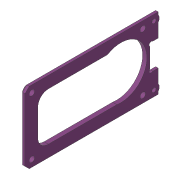
# Autodesk Inventor part: SERVO_BOTTOM_SPACER
Saved by Autodesk Inventor 2019.4 (Build 234330000, 330)
## iProperties
Created: 2019-11-13
Part Number: SERVO_BOTTOM_SPACER
Material: 一般
Document SubType Name: Modeling
Designer: y6tada
Density: 1 g/cm^3
Appearance: 滑らか - 紫
Author: y6tada
Autodesk Inventor part; units mm, degrees
ref_plane "YZ Plane" through (0, 0, 0) normal (1, 0, 0) x (0, 1, 0)
ref_plane "XZ Plane" through (0, 0, 0) normal (0, 1, 0) x (-1, 0, 0)
ref_plane "XY Plane" through (0, 0, 0) normal (0, 0, 1) x (1, 0, 0)
sketch "スケッチ1" plane through (0, 0, 0) normal (1, 0, 0) x (0, 1, 0)
  line L0 (0, 0) -> (0, 58.5) construction
  line L1 (16.75, 56.5) -> (16.75, -4)
  line L2 (16.75, -4) -> (15.5, -4)
  line L3 (6.1, -4) -> (6.1, -1.4142)
  line L4 (5.714, 0) -> (4.6858, 0) construction
  line L5 (4.6858, 0) -> (-4.6858, 0)
  line L6 (-6.1, 0) -> (-6.1, -1.4142) construction
  line L7 (-6.1, -4) -> (-12.5, -4)
  line L8 (-16.75, -4) -> (-16.75, 56.5)
  arc A0 (-4.6858, 0) -> (-6.1, -1.4142) centre (-5.3929, -0.7071) ccw
  line L9 (14.75, 58.5) -> (-14.75, 58.5)
  line L10 (16.75, 56.5) -> (14.75, 58.5)
  line L11 (-16.75, 56.5) -> (-14.75, 58.5)
  line L12 (13.5, 55.25) -> (-13.5, 55.25) construction
  line L13 (-13.5, 55.25) -> (-13.5, 3.25) construction
  line L14 (-13.5, 3.25) -> (13.5, 3.25) construction
  line L15 (13.5, 3.25) -> (13.5, 55.25) construction
  line L16 (0, 29.25) -> (21.0927, 29.25) construction
  line L17 (14, -2) -> (-14, -2) construction
  arc A1 (12.5, -4) -> (15.5, -4) centre (14, -2) ccw
  line L18 (15.5, -4) -> (12.5, -4) construction
  line L19 (12.5, -4) -> (6.1, -4)
  arc A2 (-15.5, -4) -> (-12.5, -4) centre (-14, -2) ccw
  line L20 (-12.5, -4) -> (-15.5, -4) construction
  line L21 (-15.5, -4) -> (-16.75, -4)
  line L22 (6.25, 52.5) -> (-6.25, 52.5)
  line L23 (-11.25, 47.5) -> (-11.25, 12)
  line L24 (-11.25, 12) -> (11.25, 12)
  line L25 (11.25, 12) -> (11.25, 47.5)
  arc A3 (11.25, 47.5) -> (6.25, 52.5) centre (6.25, 47.5) ccw
  arc A4 (-6.25, 52.5) -> (-11.25, 47.5) centre (-6.25, 47.5) ccw
  line L26 (6.1, -1.4142) -> (6.1, -0.7071) construction
  line L27 (-4.6858, 0) -> (-6.1, 0) construction
  line L28 (-6.1, -1.4142) -> (-6.1, -4)
  line L29 (6.1, -1.4142) -> (6.1, 0) construction
  line L30 (6.1, 0) -> (4.6858, 0) construction
  arc A5 (6.1, -1.4142) -> (4.6858, 0) centre (5.3929, -0.7071) ccw
  point P0 (16.75, 58.5)
  point P1 (-6.0944, 0.0056)
  point P2 (-16.75, 58.5)
  dimension "d3" = 12.2
  dimension "d5" = 33.5
  dimension "d6" = 4
  dimension "d7" = 58.5
  dimension "d8" = 2
  dimension "d9" = 2
  dimension "d10" = 2
  dimension "d11" = 2
  dimension "d12" = 27
  dimension "d13" = 52
  dimension "d14" = 2
  dimension "d15" = 28
  dimension "d16" = 2.5
  dimension "d33" = 5
  dimension "d34" = 5.5
  dimension "d35" = 6
  dimension "d36" = 12
  dimension "d37" = 1
  constraints: 62 end point, 16 perpendicular, 15 point on circle, 8 point on line, 7 coincident, 6 centre point, 6 horizontal, 4 parallel, 4 symmetric about line, 4 tangent, 4 vertical, 3 midpoint, 2 equal radius, 1 collinear, 6 other
  measures "d3" distance between parallel lines of L6 L3
  measures "d5" distance between parallel lines of L8 L1
  measures "d6" distance between parallel lines of L2 L5
  measures "d7" distance from line of L9 L0.start
  measures "d8" distance of L1.start point (16.75, 58.5)
  measures "d9" distance of L9.start point (16.75, 58.5)
  measures "d10" distance of L8.end point (-16.75, 58.5)
  measures "d11" distance of L9.end point (-16.75, 58.5)
  measures "d12" distance of L12.start L12.end
  measures "d13" distance of L14.end L12.start
  measures "d14" distance between parallel lines of L5 L17
  measures "d15" distance of L17.start L17.end
  measures "d16" radius of A1
  measures "d33" radius of A3
  measures "d34" distance between parallel lines of L1 L25
  measures "d35" distance between parallel lines of L9 L22
  measures "d36" distance between parallel lines of L5 L24
  measures "d37" radius of A5
extrude "押し出し1" add sketch "スケッチ1" against normal blind 1.2
sketch "スケッチ2" plane through (-1.2, 0, 0) normal (1, 0, 0) x (0, 0, -1)
  line L0 (-58.5, 14.75) -> (-58.5, -14.75) construction
  line L1 (-56.5, -16.75) -> (4, -16.75) construction
  line L2 (4, 16.75) -> (-56.5, 16.75) construction
  line L3 (0, -4.6858) -> (0, 4.6858) construction
  line L4 (-0.8, 13.9287) -> (-0.8, -13.9287)
  line L5 (-2.8213, -15.95) -> (-55.6787, -15.95)
  line L6 (-57.7, -13.9287) -> (-57.7, 13.9287)
  line L7 (-55.6787, 15.95) -> (-2.8213, 15.95)
  line L8 (-1.2393, -14.9893) -> (-1.7607, -15.5107)
  line L9 (-1.2393, 14.9893) -> (-1.7607, 15.5107)
  line L10 (-56.7393, 15.5107) -> (-57.2607, 14.9893)
  line L11 (-57.2607, -14.9893) -> (-56.7393, -15.5107)
  arc A0 (-1.2393, -14.9893) -> (-0.8, -13.9287) centre (-2.3, -13.9287) ccw
  arc A1 (-2.8213, -15.95) -> (-1.7607, -15.5107) centre (-2.8213, -14.45) ccw
  arc A2 (-56.7393, -15.5107) -> (-55.6787, -15.95) centre (-55.6787, -14.45) ccw
  arc A3 (-57.7, -13.9287) -> (-57.2607, -14.9893) centre (-56.2, -13.9287) ccw
  arc A4 (-55.6787, 15.95) -> (-56.7393, 15.5107) centre (-55.6787, 14.45) ccw
  arc A5 (-57.2607, 14.9893) -> (-57.7, 13.9287) centre (-56.2, 13.9287) ccw
  arc A6 (-1.7607, 15.5107) -> (-2.8213, 15.95) centre (-2.8213, 14.45) ccw
  arc A7 (-0.8, 13.9287) -> (-1.2393, 14.9893) centre (-2.3, 13.9287) ccw
  arc A8 (-52.5, -6.25) -> (-47.5, -11.25) centre (-47.5, -6.25) ccw projected
  line L12 (-12, -11.25) -> (-47.5, -11.25) projected
  arc A9 (-11, -11.25) -> (-6, -6.25) centre (-11, -6.25) ccw projected
  line L13 (-12, 11.25) -> (-12, -11.25) projected
  arc A10 (-6, 6.25) -> (-11, 11.25) centre (-11, 6.25) ccw projected
  line L14 (-47.5, 11.25) -> (-12, 11.25) projected
  arc A11 (-47.5, 11.25) -> (-52.5, 6.25) centre (-47.5, 6.25) ccw projected
  line L15 (-52.5, -6.25) -> (-52.5, 6.25) projected
  point P0 (0, 0)
  point P1 (-0.8, -14.55)
  point P2 (-2.2, -15.95)
  point P3 (-0.8, -15.95)
  point P4 (-0.8, 14.55)
  point P5 (-2.2, 15.95)
  point P6 (-0.8, 15.95)
  point P7 (-56.3, 15.95)
  point P8 (-57.7, 14.55)
  point P9 (-57.7, 15.95)
  point P10 (-57.7, -14.55)
  point P11 (-56.3, -15.95)
  point P12 (-57.7, -15.95)
  point P13 (52.5, -6.25)
  point P14 (47.5, -11.25)
  point P15 (47.5, 11.25)
  point P16 (52.5, 6.25)
  dimension "d38" = 1.4
  dimension "d39" = 1.4
  dimension "d40" = 1.4
  dimension "d41" = 1.4
  dimension "d42" = 1.4
  dimension "d43" = 1.4
  dimension "d44" = 1.4
  dimension "d45" = 1.4
  dimension "d46" = 1.5
  dimension "d48" = 0.8
  dimension "d50" = 0.8
  dimension "d53" = 0.8
  dimension "d54" = 0.8
  constraints: 24 point on line, 16 end point, 16 point on circle, 16 tangent, 8 centre point, 7 equal radius, 4 parallel, 4 other
  measures "d38" distance of point (-0.8, -14.55) point (-0.8, -15.95)
  measures "d39" distance of point (-2.2, -15.95) point (-0.8, -15.95)
  measures "d40" distance of point (-0.8, 14.55) point (-0.8, 15.95)
  measures "d41" distance of point (-2.2, 15.95) point (-0.8, 15.95)
  measures "d42" distance of point (-56.3, 15.95) point (-57.7, 15.95)
  measures "d43" distance of point (-57.7, 14.55) point (-57.7, 15.95)
  measures "d44" distance of point (-57.7, -14.55) point (-57.7, -15.95)
  measures "d45" distance of point (-56.3, -15.95) point (-57.7, -15.95)
  measures "d46" radius of A0
  measures "d48" distance between parallel lines of L1 L5
  measures "d50" distance between parallel lines of L2 L7
  measures "d53" distance between parallel lines of L6 L0
  measures "d54" distance between parallel lines of L3 L4
extrude "押し出し2" add sketch "スケッチ2" against normal blind 0.8
hole "穴1" at (0, 13.5, 55.25) at (0, -13.5, 55.25) at (0, -13.5, 3.25) at (0, 13.5, 3.25) direction (-1, 0, 0) diameter 2.6 end through all clearance for "Countersunk Raised Head Screw ISO 2010/7047" size "M2.5" standard "ISO"
hole "穴2" at (0, 14, -2) at (0, -14, -2) direction (-1, 0, 0) diameter 2 end through all
sketch "スケッチ3" plane through (0, 0, 0) normal (1, 0, 0) x (0, 0, -1)
  circle A0 centre (-13.5, 0.8) radius 12.2
  line L0 (4, 16.75) -> (-56.5, 16.75) projected
  line L1 (0, -4.6858) -> (0, 4.6858) projected
  point P0 (0, 0)
  dimension "d55" = 24.4
  dimension "d56" = 15.95
  dimension "d57" = 13.5
  constraints: 1 centre point
  measures "d55" diameter of A0
  measures "d56" distance from line of L0 A0.centre
  measures "d57" distance from line of L1 A0.centre
extrude "押し出し3" cut sketch "スケッチ3" against normal blind 10
equation "\"d9\" = d8"
equation "\"d11\" = d10"
equation "\"d40\" = d38"
equation "\"d41\" = d40"
equation "\"d42\" = d38"
equation "\"d43\" = d42"
equation "\"d44\" = d38"
equation "\"d45\" = d44"
